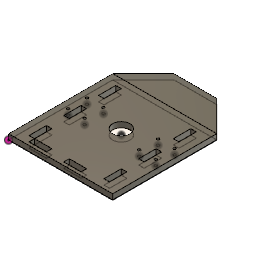
Base (Autodesk Fusion 360 design; units mm, degrees)
Autodesk Fusion 360 part; units mm, degrees
sketch "Sketch1" plane through (0, 0, 0) normal (0, 1, 0) x (1, 0, 0)
  line L0 (0, 0) -> (120, 0)
  line L1 (120, 0) -> (120, 120)
  line L2 (120, 120) -> (0, 120)
  line L3 (0, 120) -> (0, 0)
  line L4 (0, 120) -> (35.3553, 155.3553)
  line L5 (120, 120) -> (84.6447, 155.3553)
  line L6 (35.3553, 155.3553) -> (84.6447, 155.3553)
  circle A0 centre (60, 70) radius 10
  circle A1 centre (9.5, 59.15) radius 1.5
  circle A2 centre (28.55, 59.15) radius 1.5
  circle A3 centre (28.55, 80.85) radius 1.5
  circle A4 centre (9.5, 80.85) radius 1.5
  circle A5 centre (110.5, 80.85) radius 1.5
  circle A6 centre (110.5, 59.15) radius 1.5
  circle A7 centre (91.45, 59.15) radius 1.5
  circle A8 centre (91.45, 80.85) radius 1.5
  line L7 (13.65, 110) -> (20, 110)
  line L8 (20, 110) -> (20, 90)
  line L9 (20, 90) -> (13.65, 90)
  line L10 (13.65, 90) -> (13.65, 110)
  line L11 (20, 50) -> (13.65, 50)
  line L12 (13.65, 50) -> (13.65, 70)
  line L13 (13.65, 70) -> (20, 70)
  line L14 (20, 70) -> (20, 50)
  line L15 (20, 10) -> (13.65, 10)
  line L16 (13.65, 10) -> (13.65, 30)
  line L17 (13.65, 30) -> (20, 30)
  line L18 (20, 30) -> (20, 10)
  line L19 (20, 10) -> (40, 10)
  line L20 (40, 10) -> (40, 3.65)
  line L21 (40, 3.65) -> (20, 3.65)
  line L22 (20, 3.65) -> (20, 10)
  line L23 (60, 10) -> (80, 10)
  line L24 (80, 10) -> (80, 3.65)
  line L25 (80, 3.65) -> (60, 3.65)
  line L26 (60, 3.65) -> (60, 10)
  line L27 (100, 30) -> (106.35, 30)
  line L28 (106.35, 30) -> (106.35, 10)
  line L29 (106.35, 10) -> (100, 10)
  line L30 (100, 10) -> (100, 30)
  line L31 (106.35, 50) -> (100, 50)
  line L32 (100, 50) -> (100, 70)
  line L33 (100, 70) -> (106.35, 70)
  line L34 (106.35, 70) -> (106.35, 50)
  line L35 (106.35, 90) -> (100, 90)
  line L36 (100, 90) -> (100, 110)
  line L37 (100, 110) -> (106.35, 110)
  line L38 (106.35, 110) -> (106.35, 90)
  dimension "d1" = 120
  dimension "d2" = 120
  dimension "d3" = 50
  dimension "d4" = 45
  dimension "d5" = 50
  dimension "d6" = 45
  dimension "d7" = 20
  dimension "d8" = 70
  dimension "d9" = 60
  dimension "d10" = 3
  dimension "d11" = 3
  dimension "d12" = 9.5
  dimension "d13" = 19.05
  dimension "d14" = 10.85
  dimension "d15" = 10.85
  dimension "d16" = 3
  dimension "d17" = 3
  dimension "d18" = 21.7
  dimension "d19" = 21.7
  dimension "d20" = 9.5
  dimension "d21" = 19.05
  dimension "d22" = 3
  dimension "d23" = 3
  dimension "d24" = 19.05
  dimension "d25" = 3
  dimension "d26" = 3
  dimension "d27" = 21.7
  dimension "d28" = 21.7
  dimension "d29" = 19.05
  dimension "d30" = 9.5
  dimension "d78" = 9.5
  dimension "d104" = 10
  dimension "d110" = 20
  dimension "d111" = 6.35
  dimension "d112" = 20
  dimension "d113" = 10
  dimension "d114" = 20
  dimension "d115" = 6.35
  dimension "d116" = 20
  dimension "d118" = 20
  dimension "d119" = 6.35
  dimension "d120" = 20
  dimension "d121" = 20
  dimension "d122" = 6.35
  dimension "d123" = 20
  dimension "d124" = 6.35
  dimension "d125" = 20
  dimension "d126" = 20
  dimension "d127" = 10
  dimension "d128" = 20
  dimension "d129" = 6.35
  dimension "d130" = 20
  dimension "d131" = 10
  dimension "d132" = 20
  dimension "d133" = 6.35
  dimension "d134" = 20
  dimension "d135" = 20
  dimension "d136" = 6.35
  dimension "d137" = 20
  dimension "d138" = 20
  dimension "d139" = 10
  dimension "d140" = 10.85
  dimension "d141" = 10.85
  dimension "d148" = 35.3553
  measures "d4" angle of L2 L4
  measures "d6" angle of L2 L5
  measures "d7" diameter of A0
  measures "d10" diameter of A1
  measures "d11" diameter of A2
  measures "d13" distance of L0.start
  measures "d15" distance of L0.start
  measures "d16" diameter of A3
  measures "d17" diameter of A4
  measures "d21" distance of L0.start
  measures "d22" diameter of A7
  measures "d23" diameter of A6
  measures "d25" diameter of A5
  measures "d26" diameter of A8
  measures "d111" distance of L0.start
  measures "d112" distance of L3 L8
  measures "d113" distance of L2 L7
  measures "d115" distance of L0.start
  measures "d116" distance of L3 L14
  measures "d118" distance of L0.start
  measures "d120" distance of L3 L18
  measures "d121" distance of L11 L17
  measures "d126" distance of L20 L26
  measures "d127" distance of L0 L23
  measures "d128" distance of L0.start
  measures "d130" distance of L1 L30
  measures "d131" distance of L0 L29
  measures "d134" distance of L27 L31
  measures "d135" distance of L1 L32
  measures "d138" distance of L1 L36
  measures "d139" distance of L2 L37
  measures "d148" distance of L2 L6
extrude "Extrude4" add sketch "Sketch1" along normal blind 6.35 makes body 1
extrude "Extrude3" add sketch "Sketch1" along normal blind 6.35 separate body contours L0 L1 L2 L3 makes body 2
extrude "Extrude1" add sketch "Sketch1" along normal blind 6.35 separate body contours L0 L1 L2 L3 | L2 L4 L5 L6 | L7 L8 L9 L10 | L11 L12 L13 L14 | L15 L16 L17 L18 | L19 L20 L21 L22 | L23 L24 L25 L26 | L27 L28 L29 L30 | L31 L32 L33 L34 | L35 L36 L37 L38 makes body 3
extrude "Extrude5" cut sketch "Sketch1" along normal blind 6.35 contours L7 L8 L9 L10 | L11 L12 L13 L14 | L15 L16 L17 L18 | L19 L20 L21 L22 | L23 L24 L25 L26 | L27 L28 L29 L30 | L31 L32 L33 L34 | L35 L36 L37 L38 bodies 3
extrude "Extrude2" [suppressed]
